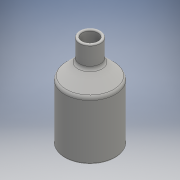
# Autodesk Inventor part: tailpipe
Saved by Autodesk Inventor 2016 (Build 200138000, 138)
## iProperties
Created: 2015-08-17
Part Number: tailpipe
Material: Generic
Document SubType Name: Modeling
Density: 1 g/cm^3
Appearance: Default
Autodesk Inventor part; units mm, degrees
ref_plane "YZ Plane" through (0, 0, 0) normal (1, 0, 0) x (0, 1, 0)
ref_plane "XZ Plane" through (0, 0, 0) normal (0, 1, 0) x (-1, 0, 0)
ref_plane "XY Plane" through (0, 0, 0) normal (0, 0, 1) x (1, 0, 0)
sketch "Sketch1" plane through (0, 0, 0) normal (0, 1, 0) x (-1, 0, 0)
  line L0 (10, 1.9794) -> (10, -18.0206)
  line L1 (10, -18.0206) -> (24.1421, -32.1628)
  line L2 (24.1421, -32.1628) -> (24.1421, -87.1628)
  line L3 (0, 0) -> (0, -84.1421)
  dimension "d0" = 20
  dimension "d1" = 20
  dimension "d2" = 135
  dimension "d3" = 55
  dimension "d5" = 5.6715
  dimension "d6" = 53.826
  dimension "d29" = 20
  constraints: 8 end point, 2 vertical, 1 parallel
  measures "d0" distance of L0.start L0.end
  measures "d1" distance of L0.end L1.end
  measures "d2" angle of L1 L0
  measures "d3" distance of L1.end L2.end
  measures "d5" distance from line of L3.start L1
  measures "d6" distance from line of L3.end L1
  measures "d29" diameter of L0 L3
surface revolve "RevolutionSrf2" sketch "Sketch1" angle 360 about axis through (0, 0, 0) along (0, 0, -1) shown no curves L0 L1 L2
thicken "Thicken2" operation new thickness 2.5 both sides no extend neighbours no toward (0.9870503, 0.1604113, 0) faces at (-9.8705, -1.6041, -4.6873) (-11.7544, -17.4014, -29.0201) (-23.8295, -3.8727, -68.8295)
fillet "Fillet1" radius 1.25 2 edges at (21.6421, 0, -87.1628) (24.1421, 0, -87.1628)
fillet "Fillet2" radius 1.25 1 edges at (21.6421, 0, -33.1983)
fillet "Fillet3" radius 1.25 1 edges at (7.5, 0, -19.0562)
fillet "Fillet4" radius 1.25 2 edges at (10, 0, 1.9794) (7.5, 0, 1.9794)
fillet "Fillet5" radius 5 2 edges at (10, 0, -18.0206) (24.1421, 0, -32.1628)
body "Solid2"
body "Srf2"
